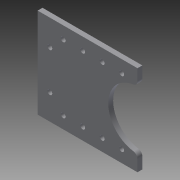
# Autodesk Inventor part: AX12_gabarit
Saved by Autodesk Inventor 2014 (Build 180170000, 170)
## iProperties
Created: 2014-01-10
Part Number: AX12_gabarit
Material: Générique
Document SubType Name: Modeling
Designer: helly
Density: 1 g/cm^3
Appearance: Par défaut
Author: helly
Autodesk Inventor part; units mm, degrees
ref_plane "YZ Plane" through (0, 0, 0) normal (1, 0, 0) x (0, 1, 0)
ref_plane "XZ Plane" through (0, 0, 0) normal (0, 1, 0) x (-1, 0, 0)
ref_plane "XY Plane" through (0, 0, 0) normal (0, 0, 1) x (1, 0, 0)
sketch "Esquisse1" plane through (0, 0, 0) normal (0, 1, 0) x (-1, 0, 0)
  line L0 (0, 0) -> (36, 0) construction
  line L1 (36, 0) -> (36, 8) construction
  line L2 (0, 0) -> (0, 13.5) construction
  line L3 (0, 13.5) -> (6.5, 13.5) construction
  line L4 (6.5, 13.5) -> (14.5, 13.5) construction
  line L5 (14.5, 13.5) -> (22.5, 13.5) construction
  line L6 (22.5, 13.5) -> (30.5, 13.5) construction
  circle A0 centre (6.5, 13.5) radius 1
  circle A1 centre (14.5, 13.5) radius 1
  circle A2 centre (22.5, 13.5) radius 1
  circle A3 centre (30.5, 13.5) radius 1
  circle A4 centre (36, 8) radius 1
  circle A5 centre (6.5, -13.5) radius 1
  circle A6 centre (14.5, -13.5) radius 1
  circle A7 centre (22.5, -13.5) radius 1
  circle A8 centre (30.5, -13.5) radius 1
  circle A9 centre (36, -8) radius 1
  line L7 (6.5, 13.5) -> (6.5, 18.5) construction
  line L8 (36, 8) -> (41, 8) construction
  circle A10 centre (0, 0) radius 12 construction
  line L9 (0, 18.5) -> (41, 18.5)
  line L10 (41, 18.5) -> (41, -18.5)
  line L11 (41, -18.5) -> (0, -18.5)
  line L12 (6.5, -13.5) -> (6.5, -18.5) construction
  line L13 (0, 18.5) -> (0, 12)
  line L14 (0, 0) -> (0, -18.5) construction
  line L15 (0, -12) -> (0, -18.5)
  arc A11 (0, -12) -> (0, 12) centre (0, 0) ccw
  dimension "d23" = 36
  dimension "d24" = 8
  dimension "d25" = 13.5
  dimension "d26" = 6.5
  dimension "d27" = 8
  dimension "d28" = 8
  dimension "d29" = 8
  dimension "d30" = 2
  dimension "d31" = 5
  dimension "d33" = 24
  constraints: 32 end point, 12 centre point, 7 coincident, 7 perpendicular, 5 collinear, 5 point on line, 5 symmetric about line, 4 equal radius, 4 point on circle, 3 parallel, 2 equal length, 1 horizontal, 5 other
  measures "d23" distance of L0.start L0.end
  measures "d24" distance of L0.end L1.end
  measures "d25" distance of L0.start L2.end
  measures "d26" distance of L2.end L3.end
  measures "d27" distance of L3.end L4.end
  measures "d28" distance of L4.end L5.end
  measures "d29" distance of L5.end L6.end
  measures "d30" diameter of A0
  measures "d31" distance of L7.start L7.end
  measures "d33" diameter of A10
extrude "Extrusion2" add sketch "Esquisse1" along normal blind 2
fillet "Congé1" radius 2 1 edges at (0, 1, 12)
fillet "Congé2" radius 2 1 edges at (0, 1, -12)
